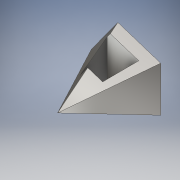
# Autodesk Inventor part: Пирамида Модель
Saved by Autodesk Inventor 2019 (Build 230136000, 136)
## iProperties
Created: 2020-03-27
Part Number: Пирамида Модель
Material: Сталь, высокопрочная, низколегированная
Document SubType Name: Modeling
Designer: Ivan
Mass: 558.216 g
Surface Area: 182.553 cm^2
Volume: 71.1103 cm^3
Density: 7.85 g/cm^3
Appearance: Сталь — полированная
Author: Ivan
Autodesk Inventor part; units mm, degrees
ref_plane "YZ Plane" through (0, 0, 0) normal (1, 0, 0) x (0, 1, 0)
ref_plane "XZ Plane" through (0, 0, 0) normal (0, 1, 0) x (-1, 0, 0)
sketch "Эскиз1" plane through (0, 0, 0) normal (0, 0, 1) x (1, 0, 0)
  line L0 (34.3832, 24.9809) -> (34.3832, -24.9809)
  line L1 (34.3832, -24.9809) -> (-13.1332, -40.4199)
  line L2 (-13.1332, -40.4199) -> (-42.5, 0)
  line L3 (-42.5, 0) -> (-13.1332, 40.4199)
  line L4 (-13.1332, 40.4199) -> (34.3832, 24.9809)
  point P0 (0, 0)
  point P1 (0, 0)
  dimension "d2" = 76.8832
  constraints: 10 end point, 1 coincident, 1 vertical, 11 other
  measures "d2" distance from line of L0 L2.end
ref_plane "РабПлоскость1" through (0, 0, 80) normal (0, 0, 1) x (1, 0, 0)
sketch "Эскиз2" plane through (0, 0, 80) normal (0, 0, 1) x (1, 0, 0)
  point P0 (0, 0)
  point P1 (0, 0)
loft "Лофт1" add profiles "Эскиз1" section 2 point at (0, 0, 80)
sketch "Эскиз3" plane through (0, 0, 0) normal (0, 1, 0) x (-1, 0, 0)
  line L0 (15, 10) -> (15, 40)
  line L1 (15, 40) -> (-10, 40)
  line L2 (-10, 40) -> (-20, 10)
  line L3 (-20, 10) -> (15, 10)
  point P0 (0, 0)
  dimension "d10" = 35
  dimension "d11" = 25
  dimension "d12" = 30
  dimension "d13" = 15
  dimension "d14" = 10
  constraints: 8 end point, 2 horizontal, 1 vertical
  measures "d10" distance of L2.end L0.start
  measures "d11" distance of L1.end L0.end
  measures "d12" distance between parallel lines of L3 L1
  measures "d13" distance from line of point (0, 0) L0
  measures "d14" distance from line of point (0, 0) L3
extrude "Выдавливание1" cut sketch "Эскиз3" along normal through all both and the other way through all
